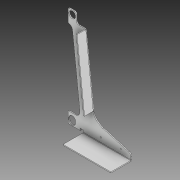
# Autodesk Inventor part: FE-110-006 Side Holder
Saved by Autodesk Inventor 2021 (Build 250183000, 183)
## iProperties
Created: 2021-01-11
Part Number: FE-110-006 Side Holder
Material: Aluminum 6061
Document SubType Name: Sheet Metal
Density: 2.7 g/cm^3
Sheet Metal Rule: Default
Appearance: Aluminum - Dark
Autodesk Inventor part; units mm, degrees
ref_plane "YZ Plane" through (0, 0, 0) normal (1, 0, 0) x (0, 1, 0)
ref_plane "XZ Plane" through (0, 0, 0) normal (0, 1, 0) x (-1, 0, 0)
ref_plane "XY Plane" through (0, 0, 0) normal (0, 0, 1) x (1, 0, 0)
sketch "Sketch1" plane through (0, 0, 0) normal (0, 0, 1) x (1, 0, 0)
  circle A0 centre (0, 229.3938) radius 16.9545
  line L0 (0, -229.3938) -> (0, -237.0392) construction
  line L1 (-16.9545, -229.3937) -> (-16.9545, -237.0391)
  line L2 (16.9545, -237.0392) -> (16.9545, -229.3938)
  arc A1 (16.9545, -229.3938) -> (-16.9545, -229.3937) centre (0, -229.3938) ccw
  arc A2 (-16.9545, -237.0391) -> (16.9545, -237.0392) centre (0, -237.0392) ccw
  line L3 (63.7794, 199.9298) -> (20.701, 199.9298)
  line L4 (20.701, 199.9298) -> (20.701, 250.3996)
  line L5 (20.701, 250.3996) -> (-20.574, 250.3996)
  line L6 (-20.574, 250.3996) -> (-20.574, 183.0357)
  arc A3 (1.5167, 163.2505) -> (-20.574, 183.0357) centre (-20.574, 160.8107) ccw
  line L7 (-20.574, 183.0357) -> (22.7676, 183.0357) construction
  line L8 (1.5167, 163.2505) -> (41.6845, -200.4378)
  line L9 (63.7794, 199.9298) -> (101.2188, -139.0548)
  line L10 (41.6845, -200.4378) -> (-20.574, -200.4378)
  line L11 (-20.574, -200.4378) -> (-20.574, -257.6132)
  line L12 (-20.574, -257.6132) -> (40.5384, -257.6132)
  line L13 (40.5384, -257.6132) -> (40.5384, -246.107)
  line L14 (40.5384, -246.107) -> (42.926, -246.107)
  line L15 (42.926, -246.107) -> (42.926, -247.3008)
  line L16 (42.926, -247.3008) -> (55.626, -247.3008)
  line L17 (55.626, -247.3008) -> (55.626, -257.6132)
  line L18 (55.626, -257.6132) -> (296.926, -257.6132)
  line L19 (296.926, -257.6132) -> (296.926, -232.2132)
  line L20 (296.926, -232.2132) -> (154.2472, -190.7527)
  arc A4 (104.0038, -143.9092) -> (154.2472, -190.7527) centre (175.5103, -117.5795) ccw
  line L21 (101.2188, -139.0548) -> (91.3222, -140.1478)
  line L22 (91.3222, -140.1478) -> (91.8855, -145.2476)
  line L23 (91.8855, -145.2476) -> (104.0038, -143.9092)
  circle A5 centre (55.626, -138.5126) radius 3.302
  circle A6 centre (55.626, -62.3126) radius 3.302
  circle A7 centre (55.626, 13.8874) radius 3.302
  circle A8 centre (55.626, 90.0874) radius 3.302
  circle A9 centre (55.626, 166.2874) radius 3.302
  circle A10 centre (246.126, -235.3882) radius 3.302
  circle A11 centre (144.526, -235.3882) radius 3.302
  point P0 (0, 0)
  point P1 (0, -233.2165)
  dimension "d0" = 33.909
  dimension "d1" = 458.7875
  dimension "d2" = 7.6454
  dimension "d3" = 229.3938
  dimension "d4" = 21.0058
  dimension "d5" = 20.574
  dimension "d6" = 20.701
  dimension "d7" = 22.225
  dimension "d8" = 65.913
  dimension "d9" = 6.303
  dimension "d10" = 43.0784
  dimension "d11" = 50.4698
  dimension "d12" = 28.956
  dimension "d13" = 20.574
  dimension "d14" = 20.574
  dimension "d15" = 341.0458
  dimension "d16" = 61.1124
  dimension "d17" = 1.1938
  dimension "d18" = 2.3876
  dimension "d19" = 10.3124
  dimension "d20" = 15.0876
  dimension "d21" = 241.3
  dimension "d22" = 9.9568
  dimension "d23" = 5.1308
  dimension "d24" = 2.2352
  dimension "d25" = 25.4
  dimension "d26" = 76.2
  dimension "d55" = 119.1006
  dimension "d56" = 76.2
  dimension "d57" = 6.604
  dimension "d60" = 76.2
  dimension "d65" = 101.6
  dimension "d66" = 50.8
  dimension "d67" = 22.225
  measures "d0" diameter of A0
  measures "d1" distance of A0.centre L0.start
  measures "d2" distance of L0.start L0.end
  measures "d3" distance of point (0, 0) A0.centre
  measures "d4" distance from line of A0.centre L5
  measures "d5" distance from line of A0.centre L6
  measures "d6" distance from line of L4 A0.centre
  measures "d7" radius of A3
  measures "d8" distance between parallel lines of L8 L9
  measures "d9" angle of L4 L9
  measures "d10" distance of L3.start L3.end
  measures "d11" distance between parallel lines of L5 L3
  measures "d12" distance from line of L10 L0.start
  measures "d13" distance from line of L12 L0.end
  measures "d14" distance from line of L11 L0.end
  measures "d15" distance of L3.start L9.end
  measures "d16" distance of L11.end L12.end
  measures "d17" distance between parallel lines of L14 L16
  measures "d18" distance of L13.end L14.end
  measures "d19" distance between parallel lines of L12 L16
  measures "d20" distance between parallel lines of L17 L13
  measures "d21" distance of L17.end L18.end
  measures "d22" distance of L9.end L21.end
  measures "d23" distance of L21.end L22.end
  measures "d24" distance from line of L9 L23.end
  measures "d25" distance of L18.end L19.end
  measures "d26" radius of A4
  measures "d55" distance from line of L12 A5.centre
  measures "d56" distance from line of A5.centre L11
  measures "d57" diameter of A5
  measures "d60" distance of A5.centre A6.centre
  measures "d65" distance of A11.centre A10.centre
  measures "d66" distance from line of L19 A10.centre
  measures "d67" distance from line of A10.centre L18
extrude "Plate1" add sketch "Sketch1" along normal blind 4.826
sketch "Sketch2" plane through (296.926, -259.6706, 6.8834) normal (0, -1, 0) x (1, 0, 0)
  line L0 (-241.3, 0) -> (0, 0)
  line L1 (0, 0) -> (0, 99.5426)
  line L2 (0, 99.5426) -> (-241.3, 99.5426)
  line L3 (-241.3, 99.5426) -> (-241.3, 0)
  constraints: 6 end point, 1 horizontal, 1 perpendicular, 1 vertical
edge flange "Flange1" height 106.426 angle 90 thickness 4.826 bend radius 2.0574 thickness toward (0, -1, 0) relief tear relief width 4.826 relief depth 2.413 edges at (176.276, -257.6132, 4.826) wall of the first edge with corners at (55.626, -259.6706, 6.8834) (296.926, -259.6706, 6.8834) (296.926, -259.6706, 106.426) (55.626, -259.6706, 106.426)
bend "Bend1"
corner "Corner1"
sketch "Sketch3" plane through (65.8244, 200.1556, 6.8834) normal (0.9939561, 0.1097783, 0) x (-0.1097783, 0.9939561, 0)
  line L0 (-341.0458, 0) -> (0, 0)
  line L1 (0, 0) -> (0, 43.9166)
  line L2 (0, 43.9166) -> (-341.0458, 43.9166)
  line L3 (-341.0458, 43.9166) -> (-341.0458, 0)
  constraints: 6 end point, 1 horizontal, 1 perpendicular, 1 vertical
edge flange "Flange2" height 50.8 angle 90 thickness 4.826 bend radius 2.0574 thickness toward (0.9939561, 0.1097783, 0) relief tear relief width 4.826 relief depth 2.413 edges at (82.4991, 30.4375, 4.826) wall of the first edge with corners at (103.2638, -138.8289, 6.8834) (65.8244, 200.1556, 6.8834) (65.8244, 200.1556, 50.8) (103.2638, -138.8289, 50.8)
bend "Bend2"
corner "Corner2"
fillet "Corner Round1" radius 15.875 1 edges at (296.926, -232.2132, 2.413)
fillet "Corner Round1" radius 1.1938 2 edges at (42.926, -246.107, 2.413) (40.5384, -246.107, 2.413)
fillet "Corner Round1" radius 6.35 2 edges at (-20.574, -257.6132, 2.413) (-20.574, 250.3996, 2.413)
fillet "Corner Round1" radius 3.175 2 edges at (-20.574, -200.4378, 2.413) (-20.574, 183.0357, 2.413)
fillet "Corner Round1" radius 22.225 1 edges at (41.6845, -200.4378, 2.413)
fillet "Corner Round1" radius 12.7 2 edges at (20.701, 250.3996, 2.413) (20.701, 199.9298, 2.413)
fillet "Corner Round1" radius 2.5654 2 edges at (91.8855, -145.2476, 2.413) (91.3222, -140.1478, 2.413)
equation "\"d3\" = 0.5 * d1"
equation "\"d18\" = 2 * d17"
equation "\"d27\" = Thickness"
equation "\"d28\" = BendReliefWidth"
equation "\"d29\" = BendReliefDepth"
equation "\"d30\" = MinimumRemnant"
equation "\"d31\" = TransitionRadius"
equation "\"d34\" = BendRadius"
equation "\"d35\" = CornerReliefSize"
equation "\"d36\" = GapSize"
equation "\"d37\" = JacobiRadiusSize"
equation "\"d38\" = BendReliefWidth"
equation "\"d39\" = BendReliefDepth"
equation "\"d40\" = MinimumRemnant"
equation "\"d41\" = TransitionRadius"
equation "\"d44\" = BendRadius"
equation "\"d45\" = CornerReliefSize"
equation "\"d46\" = GapSize"
equation "\"d47\" = JacobiRadiusSize"
equation "\"BendReliefWidth\" = Thickness"
equation "\"BendReliefDepth\" = 0.5 * Thickness"
equation "\"CornerReliefSize\" = 4 * Thickness"
equation "\"MinimumRemnant\" = 2 * Thickness"
equation "\"TransitionRadius\" = BendRadius"
equation "\"JacobiRadiusSize\" = BendRadius"
equation "\"GapSize\" = Thickness"
equation "\"Thickness\" = 4.826"
equation "\"BendRadius\" = 2.0574"
body "Solid1"
